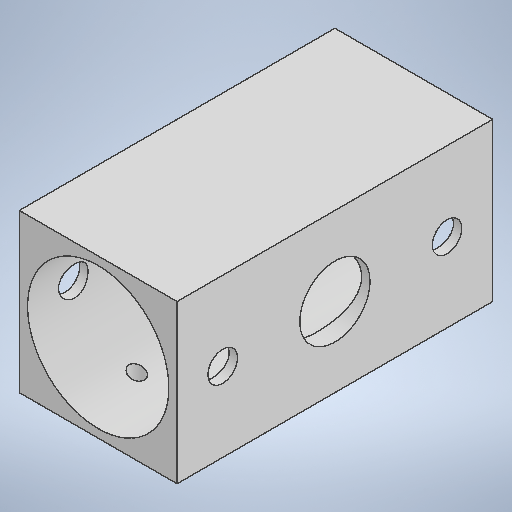
# Autodesk Inventor part: Bohrschablone_Unten
Saved by Autodesk Inventor 2026.2 (Build 302298000, 298)
## iProperties
Created: 2026-03-24
Part Number: Bohrschablone_Unten
Material: Generic
Document SubType Name: Modeling
Designer: Paco Ariel
Density: 1 g/cm^3
Appearance: Default
Author: Paco Ariel
Autodesk Inventor part; units mm, degrees
ref_plane "YZ Plane" through (0, 0, 0) normal (1, 0, 0) x (0, 1, 0)
ref_plane "XZ Plane" through (0, 0, 0) normal (0, 1, 0) x (-1, 0, 0)
ref_plane "XY Plane" through (0, 0, 0) normal (0, 0, 1) x (1, 0, 0)
sketch "Sketch1" plane through (0, 0, 0) normal (0, 0, 1) x (1, 0, 0)
  line L0 (-22.5, 22.5) -> (22.5, 22.5)
  line L1 (22.5, 22.5) -> (22.5, -22.5)
  line L2 (22.5, -22.5) -> (-22.5, -22.5)
  line L3 (-22.5, -22.5) -> (-22.5, 22.5)
  line L4 (-22.5, 22.5) -> (22.5, -22.5) construction
  line L5 (22.5, 22.5) -> (-22.5, -22.5) construction
  circle A0 centre (0, 0) radius 20.125
  dimension "d0" = 45
  dimension "d1" = 45
  dimension "d2" = 40.25
  constraints: 12 end point, 2 midpoint, 2 parallel, 1 centre point, 1 coincident, 1 horizontal, 1 perpendicular
  measures "d0" distance of L1.end L2.end
  measures "d1" distance of L0.end L1.end
  measures "d2" diameter of A0
extrude "Extrusion1" add sketch "Sketch1" against normal blind 90
sketch "Sketch2" plane through (22.5, -22.5, 0) normal (1, 0, 0) x (0, 0, -1)
  line L0 (0, 22.5) -> (13, 22.5)
  line L1 (13, 22.5) -> (77, 22.5)
  dimension "d5" = 13
  dimension "d6" = 64
  constraints: 4 end point, 2 coincident, 1 horizontal, 1 point on line
  measures "d5" distance of L0.start L0.end
  measures "d6" distance of L0.end L1.end
hole "Hole1" at (22.5, 0, -13) at (22.5, 0, -77) direction (-1, 0, 0) diameter 8.4 end through all
sketch "Sketch3" plane through (22.5, -22.5, 0) normal (1, 0, 0) x (0, 0, -1)
  line L0 (0, 22.5) -> (45, 22.5)
  dimension "d14" = 45
  constraints: 2 end point, 1 coincident, 1 horizontal
  measures "d14" distance of L0.start L0.end
hole "Hole2" at (22.5, 0, -45) direction (-1, 0, 0) diameter 20 end through all
sketch "Sketch4" plane through (-22.5, -22.5, 0) normal (0, -1, 0) x (1, 0, 0)
  line L0 (22.5, 0) -> (22.5, -18)
  line L1 (15.5, -18) -> (29.5, -18)
  dimension "d22" = 18
  dimension "d30" = 14
  constraints: 4 end point, 2 coincident, 1 horizontal, 1 vertical
  measures "d22" distance of L0.start L0.end
  measures "d30" distance of L1.start L1.end
hole "Hole3" at (-7, -22.5, -18) at (7, -22.5, -18) direction (0, 1, 0) diameter 4.3 depth 8 tip angle 118
body "Solid1"
